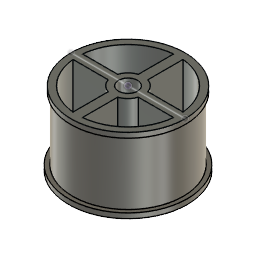
parameterized_tire_and_rim (Autodesk Fusion 360 archive; units mm, degrees)
design "Tire and Rim"
part number: 2026-01-23-22-31-03-198
Autodesk Fusion 360 part; units mm, degrees
sketch "Sketch1" plane through (0, 0, 0) normal (0, 0, 1) x (1, 0, 0)
  circle A0 centre (0, 0) radius 9.9
  circle A1 centre (0, 0) radius 8.75
  dimension "outerDiameter" = 19.8
  dimension "innerDiameter" = 17.5
  constraint coincident A0.centre A1.centre
  measures "outerDiameter" diameter of A0
  measures "innerDiameter" diameter of A1
extrude "Extrude1" add sketch "Sketch1" along normal blind 10 makes body 1
fillet "Fillet1" radius 0.5 1 edges at (-9.23, -3.58, 10) on bodies 1
fillet "Fillet2" radius 0.5 1 edges at (-9.23, -3.58, 0) on bodies 1
sketch "Sketch2" plane through (0, 0, 0) normal (0, 0, 1) x (1, 0, 0)
  circle A0 centre (0, 0) radius 8.75
  line L0 (0, 2.5) -> (0.0007, 2.5)
  arc A1 (-7.9648, -0.75) -> (-0.75, -7.9648) centre (0, 0) ccw
  arc A2 (-2.3848, -0.75) -> (-0.75, -2.3848) centre (0, 0) ccw
  arc A3 (0.75, -2.3848) -> (2.3848, -0.75) centre (0, 0) ccw
  arc A4 (0.75, -7.9648) -> (7.9648, -0.75) centre (0, 0) ccw
  arc A5 (7.9641, 0.7569) -> (0.75, 7.9648) centre (0, 0) ccw
  arc A6 (-0.5, 7.9844) -> (-7.9648, 0.75) centre (0, 0) ccw
  line L1 (0.25, 2.5) -> (0.25, 2.4875)
  arc A7 (2.3827, 0.7569) -> (0.75, 2.3848) centre (0, 0) ccw
  arc A8 (-0.75, 2.3848) -> (-2.3848, 0.75) centre (0, 0) ccw
  line L2 (-0.5, 7.9844) -> (-0.5, 8)
  line L3 (-4.6, 0.75) -> (-2.3848, 0.75)
  line L4 (-4.6, 0.75) -> (-7.9648, 0.75)
  line L5 (-4.5, -0.75) -> (-2.3848, -0.75)
  line L6 (-4.5, -0.75) -> (-7.9648, -0.75)
  line L7 (-0.75, 3) -> (-0.75, 2.3848)
  line L8 (-0.75, 3) -> (-0.75, 7.9648)
  line L9 (0.75, 3) -> (0.75, 2.3848)
  line L10 (0.75, 3) -> (0.75, 7.9648)
  line L11 (3.9807, -0.75) -> (7.9648, -0.75)
  line L12 (3.9807, -0.75) -> (2.3848, -0.75)
  line L13 (4.0259, 0.7569) -> (7.9641, 0.7569)
  line L14 (4.0259, 0.7569) -> (2.3827, 0.7569)
  line L15 (-0.75, -4.9782) -> (-0.75, -2.3848)
  line L16 (-0.75, -4.9782) -> (-0.75, -7.9648)
  line L17 (0.75, -4.9563) -> (0.75, -2.3848)
  line L18 (0.75, -4.9563) -> (0.75, -7.9648)
  circle A9 centre (0, 0) radius 1.5
  dimension "rimOuterDiameter" = 17.5
  dimension "spokeThickness" = 0.25
  dimension "d69" = 3
  constraint coincident A0.centre A1.centre
  constraint concentric A0 A2
  constraint concentric A3 A4
  constraint coincident L0.start A7
  constraint concentric A1 A6
  constraint concentric A2 A8
  constraint concentric A2 A3
  constraint concentric A4 A5
  constraint concentric A5 A6
  constraint concentric A7 A8
  constraint coincident A6 L8.end
  constraint concentric A0 A9
  measures "rimOuterDiameter" diameter of A0
  measures "spokeThickness" distance of L0.start L1.start
  measures "d69" diameter of A9
sketch "Sketch4" plane through (0, 0, 0) normal (1, 0, 0) x (0, 1, 0)
extrude "Extrude4" add sketch "Sketch2" along normal blind 11.6 separate body makes body 2
move_body "Move1" bodies 1 to x (1, 0, 0) y (0, 1, 0) z (0, 0, 1) at (0, 0, 0.8)
move_body "Move6" bodies 1 2 to x (1, 0, 0) y (0, 1, 0) z (0, 0, 1) at (0, 0, -5.8)
sketch "Sketch8" plane through (0, 0, 0) normal (0, 1, 0) x (1, 0, 0)
  line L0 (8.7, 5.8) -> (8.7, -5.8)
  line L1 (8.7, -5.8) -> (9.4, -5.8)
  line L2 (8.7, 0) -> (0, 0)
  line L3 (8.7, 5.8) -> (9.4, 5.8)
  line L4 (9.4, -5) -> (9.4, -5.8)
  line L5 (9.4, 5) -> (9.4, 5.8)
  line L6 (9.05, -5.8) -> (9.05, -5)
  line L7 (9.4, -5.8) -> (9.4, -5)
  line L8 (9.4, -5) -> (8.7, -5)
  line L9 (9.4, 5.8) -> (9.4, 5)
  line L10 (9.4, 5) -> (8.7, 5)
  dimension "lipOffset" = 11.6
  dimension "d66" = 0.8
  dimension "d67" = 0.8
  constraint vertical L0
  constraint perpendicular L0 L1
  constraint midpoint L0 L2.start
  constraint coincident L2.end origin
  constraint perpendicular L0 L3
  constraint perpendicular L1 L4
  constraint perpendicular L3 L5
  constraint midpoint L1 L6.start
  constraint perpendicular L1 L7
  constraint coincident L0 L8.end
  constraint perpendicular L0 L8
  constraint coincident L8 L6.end
  constraint perpendicular L3 L9
  constraint coincident L0 L10.end
  constraint perpendicular L0 L10
  measures "lipOffset" distance of L0.start L0.end
  measures "d66" distance of L1.end L4.start
  measures "d67" distance of L3.end L5.start
revolve "Revolve2" add sketch "Sketch8" angle 360 about axis through (0, 0, 1.75) along (0, 0, 1) contours L0 L3 L5 L9 L10 | L0 L1 L6 L8 bodies 2
sketch "Sketch9" plane through (0, 0, 5.8) normal (0, 0, 1) x (-1, 0, 0)
  circle A0 centre (0, 0) radius 9.05
  circle A1 centre (0, 0) radius 1.5
  line L0 (7.9648, 0.75) -> (2.3848, 0.75)
  arc A2 (2.3848, 0.75) -> (0.75, 2.3848) centre (0, 0) ccw
  line L1 (0.75, 2.3848) -> (0.75, 7.9648)
  arc A3 (7.9648, 0.75) -> (0.75, 7.9648) centre (0, 0) ccw
  line L2 (-0.75, 7.9648) -> (-0.75, 2.3848)
  arc A4 (-0.75, 2.3848) -> (-2.3848, 0.75) centre (0, 0) ccw
  line L3 (-2.3848, 0.75) -> (-7.9648, 0.75)
  arc A5 (-0.75, 7.9648) -> (-7.9648, 0.75) centre (0, 0) ccw
  line L4 (0.75, -7.9648) -> (0.75, -2.3848)
  arc A6 (0.75, -2.3848) -> (2.3848, -0.75) centre (0, 0) ccw
  line L5 (2.3848, -0.75) -> (7.9648, -0.75)
  arc A7 (0.75, -7.9648) -> (7.9648, -0.75) centre (0, 0) ccw
  arc A8 (-7.9641, -0.7569) -> (-0.75, -7.9648) centre (0, 0) ccw
  line L6 (-7.9641, -0.7569) -> (-2.3827, -0.7569)
  arc A9 (-2.3827, -0.7569) -> (-0.75, -2.3848) centre (0, 0) ccw
  line L7 (-0.75, -2.3848) -> (-0.75, -7.9648)
  line L8 (0, 0) -> (-9.05, 0)
  line L9 (0, 0) -> (9.05, 0)
  constraint coincident A0.centre A1.centre
  constraint coincident A0 L8.end
  constraint parallel L6 L8
  constraint coincident A0 L9.end
  constraint parallel L8 L9
sketch "Sketch10" plane through (0, 0, 0) normal (0, 1, 0) x (1, 0, 0)
sketch "Sketch11" plane through (0, 0, 5.8) normal (0, 0, 1) x (-1, 0, 0)
hidden bodies 1
equation "tireWidth = 10 mm"
equation "filletAngle = 0.5 mm"
equation "otherFillet = filletAngle"
equation "rimOuterDiameter = innerDiameter"
equation "rimWidth = tireWidth + ( 2 * 0.8 ) * 1 mm"
equation "lipWidth = 0.8 mm"
equation "midlineOffset = -( 0.5 * rimWidth )"
equation "lipOffset = rimWidth"
